honda_cup_holder_holder_v2 (Autodesk Fusion 360 design; units mm, degrees)
Autodesk Fusion 360 part; units mm, degrees
note: some values were not read from the file. Set by a fixed rule: which sketch regions a step uses.
sketch "Right Rail" plane through (0, 0, 0) normal (1, 0, 0) x (0, 0, -1)
  line L0 (7.5, 117.1) -> (11, 117.1)
  line L1 (11, 127.5) -> (16, 124.55)
  line L2 (16, 120.05) -> (11, 117.1)
  line L3 (16, 124.55) -> (16, 120.05)
  line L4 (11, 127.5) -> (7.5, 127.5)
  line L5 (7.5, 127.5) -> (7.5, 117.1)
  dimension "d1" = 5
  dimension "d2" = 4.5
  dimension "d5" = 8.5
  dimension "d16" = 10.4
  dimension "d17" = 7.5
  dimension "d18" = 127.5
  constraint equal L1 L2
  constraint perpendicular L0 L5
  constraint vertical L3
  constraint equal L0 L4
  measures "d1" distance of L1.start L3
  measures "d2" distance of L1.end L2.start
  measures "d5" distance of L3 L5
  measures "d16" distance of L0 L4
  measures "d17" horizontal distance of origin L4.end
  measures "d18" distance of origin L4
sketch "Phone Holder" plane through (0, 0, 0) normal (0, 1, 0) x (1, 0, 0)
  line L0 (0, 7.5) -> (0, -122.5)
  line L1 (0, -122.5) -> (21.5, -122.5)
  line L2 (21.5, -122.5) -> (21.5, 7.5)
  line L3 (21.5, 7.5) -> (0, 7.5)
  line L4 (2, -10) -> (19.5, -10)
  line L5 (19.5, -10) -> (19.5, -105)
  line L6 (19.5, -105) -> (2, -105)
  line L7 (2, -105) -> (2, -10)
  line L8 (2, -105) -> (2, -122.5) construction
  line L9 (2, -10) -> (2, 7.5) construction
  dimension "d6" = 2
  dimension "d7" = 2
  dimension "d8" = 17.5
  dimension "d9" = 95
  dimension "d10" = 7.5
  dimension "d11" = 130
  constraint vertical L0
  constraint perpendicular L0 L1
  constraint perpendicular L1 L2
  constraint perpendicular L2 L3
  constraint horizontal L4
  constraint vertical L5
  constraint horizontal L6
  constraint vertical L7
  constraint coincident origin L0
  constraint coincident L1 L8.end
  constraint perpendicular L1 L8
  constraint coincident L3 L9.end
  constraint perpendicular L3 L9
  constraint equal L8 L9
  measures "d6" distance of L2 L5
  measures "d7" distance of L0 L7
  measures "d8" distance of L4.start L4.end
  measures "d9" distance of L4 L6
  measures "d10" distance of L3 origin
  measures "d11" distance of L1 L3
extrude "Extrude2" add sketch "Phone Holder" along normal blind 3 contours L4 L5 L6 L7 makes body 1
extrude "Extrude1" add sketch "Phone Holder" along normal blind 130 separate body makes body 2
extrude "Extrude3" add sketch "Right Rail" along normal blind 21.5 bodies 2
sketch "Spring Rail Hole" plane through (0, 0, 122.5) normal (0, 0, 1) x (1, 0, 0)
  line L0 (0, 0) -> (21.5, 0)
  line L1 (21.5, 0) -> (21.5, 130)
  line L2 (21.5, 130) -> (0, 130)
  line L3 (0, 130) -> (0, 0)
  line L4 (2.5, 127.5) -> (2.5, 116.9)
  line L5 (19, 116.9) -> (19, 127.5)
  line L6 (19, 127.5) -> (2.5, 127.5)
  line L7 (2.5, 116.9) -> (9.375, 116.9)
  line L8 (9.375, 116.9) -> (9.375, 113.9)
  line L9 (9.375, 113.9) -> (12.125, 113.9)
  line L10 (12.125, 113.9) -> (12.125, 116.9)
  line L11 (12.125, 116.9) -> (19, 116.9)
  dimension "d21" = 2.5
  dimension "d23" = 2.5
  dimension "d24" = 2.5
  dimension "d27" = 2.75
  dimension "d29" = 3
  dimension "d30" = 10.6
  constraint parallel L3 L4
  constraint horizontal L6
  constraint perpendicular L4 L7
  constraint perpendicular L7 L8
  constraint perpendicular L4 L9
  constraint perpendicular L9 L10
  constraint equal L7 L11
  constraint coincident L5.start L11.end
  constraint perpendicular L5 L11
  constraint collinear L7 L11
  measures "d21" distance of L2 L6
  measures "d23" distance of L1 L5
  measures "d24" distance of L3 L4
  measures "d27" distance of L8.end L9.end
  measures "d29" distance of L9.end L10.end
  measures "d30" distance of L5.start L5.end
extrude "Extrude4" cut sketch "Spring Rail Hole" against normal blind 15 contours L4 L5 L6 L7 L8 L9 L10 L11 bodies 2
sketch "Spting Cross" plane through (0, 0, 107.5) normal (0, 0, 1) x (1, 0, 0)
  line L0 (12.125, 116.9) -> (19, 116.9)
  line L1 (19, 116.9) -> (19, 127.5)
  line L2 (19, 127.5) -> (2.5, 127.5)
  line L3 (2.5, 127.5) -> (2.5, 116.9)
  line L4 (2.5, 116.9) -> (9.375, 116.9)
  line L5 (9.375, 116.9) -> (9.375, 113.9)
  line L6 (9.375, 113.9) -> (12.125, 113.9)
  line L7 (12.125, 113.9) -> (12.125, 116.9)
  line L8 (10.25, 124.7) -> (10.25, 122.7)
  line L9 (10.25, 122.7) -> (8.25, 122.7)
  line L10 (8.25, 122.7) -> (8.25, 121.7)
  line L11 (8.25, 121.7) -> (10.25, 121.7)
  line L12 (10.25, 121.7) -> (10.25, 119.7)
  line L13 (10.25, 119.7) -> (11.25, 119.7)
  line L14 (11.25, 119.7) -> (11.25, 121.7)
  line L15 (11.25, 121.7) -> (13.25, 121.7)
  line L16 (13.25, 121.7) -> (13.25, 122.7)
  line L17 (13.25, 122.7) -> (11.25, 122.7)
  line L18 (10.25, 124.7) -> (11.25, 124.7)
  line L19 (11.25, 124.7) -> (11.25, 122.7)
  line L20 (8.25, 122.2) -> (13.25, 122.2) construction
  line L21 (2.5, 122.2) -> (19, 122.2) construction
  dimension "d31" = 1
  dimension "d32" = 5
  constraint perpendicular L2 L8
  constraint perpendicular L8 L9
  constraint perpendicular L9 L10
  constraint perpendicular L10 L11
  constraint perpendicular L11 L12
  constraint perpendicular L12 L13
  constraint perpendicular L13 L14
  constraint perpendicular L14 L15
  constraint perpendicular L15 L16
  constraint perpendicular L16 L17
  constraint perpendicular L8 L18
  constraint perpendicular L17 L19
  constraint equal L8 L19
  constraint equal L9 L17
  constraint equal L8 L12
  constraint equal L11 L15
  constraint equal L8 L9
  constraint equal L14 L15
  constraint equal L13 L18
  constraint equal L16 L18
  constraint midpoint L10 L20.start
  constraint midpoint L16 L20.end
  constraint midpoint L3 L21.start
  constraint midpoint L1 L21.end
  constraint midpoint L20 L21
  measures "d31" distance of L8.start L18.end
  measures "d32" distance of L10 L16
extrude "Extrude5" add sketch "Spting Cross" along normal blind 7.5 contours L8 L9 L10 L11 L12 L13 L14 L15 L16 L17 L18 L19 bodies 2
sketch "Phone Holder Hole" plane through (21.5, 0, 0) normal (1, 0, 0) x (0, 0, -1)
  line L0 (-122.5, 0) -> (7.5, 0)
  line L1 (7.5, 0) -> (7.5, 117.1)
  line L2 (7.5, 117.1) -> (11, 117.1)
  line L3 (11, 117.1) -> (16, 120.05)
  line L4 (16, 120.05) -> (16, 124.55)
  line L5 (16, 124.55) -> (11, 127.5)
  line L6 (11, 127.5) -> (7.5, 127.5)
  line L7 (7.5, 127.5) -> (7.5, 130)
  line L8 (7.5, 130) -> (-122.5, 130)
  line L9 (-122.5, 130) -> (-122.5, 0)
  line L10 (-72.5, 130) -> (-72.5, 70)
  arc A0 (-72.5, 70) -> (-42.5, 70) centre (-57.5, 70) ccw
  line L11 (-42.5, 70) -> (-42.5, 130)
  line L12 (-122.5, 130) -> (-72.5, 130) construction
  line L13 (-42.5, 130) -> (7.5, 130) construction
  circle A1 centre (-97.5, 25) radius 12.5
  circle A2 centre (-17.5, 25) radius 12.5
  circle A3 centre (-57.5, 25) radius 12.5
  line L14 (-122.5, 25) -> (7.5, 25) construction
  line L15 (-122.5, 0) -> (7.5, 0) construction
  line L16 (-57.5, 70) -> (-57.5, 25) construction
  line L17 (-97.5, 25) -> (-97.5, 70) construction
  line L18 (-17.5, 25) -> (-17.5, 70) construction
  line L19 (-17.5, 70) -> (-97.5, 70) construction
  circle A4 centre (-97.5, 70) radius 53.4439 construction
  circle A5 centre (-97.5, 70) radius 12.5
  circle A6 centre (-17.5, 70) radius 12.5
  line L20 (-97.5, 70) -> (-97.5, 102.4132) construction
  line L21 (-17.5, 101.7961) -> (-97.5, 102.4132) construction
  line L22 (-17.5, 101.7961) -> (-17.5, 70) construction
  circle A7 centre (-97.5, 102.4132) radius 13.0731 construction
  circle A8 centre (-17.5, 101.7961) radius 13.7934 construction
  dimension "d35" = 30
  dimension "d36" = 60
  dimension "d47" = 40
  dimension "d48" = 40
  dimension "d49" = 25
  dimension "d50" = 25
  dimension "d51" = 25
  dimension "d52" = 25
  dimension "d53" = 25
  dimension "d54" = 25
  dimension "d55" = 45
  constraint coincident L8 L10.start
  constraint perpendicular L8 L10
  constraint tangent L10 A0
  constraint coincident L8 L11.end
  constraint tangent A0 L11
  constraint perpendicular L8 L11
  constraint coincident L8.end L9.start
  constraint coincident L7.end L8.start
  constraint equal L12 L13
  constraint coincident L9 L14.start
  constraint coincident L1 L14.end
  constraint perpendicular L1 L14
  constraint coincident A1.centre L14
  constraint coincident A3.centre L14
  constraint coincident A2.centre L14
  constraint coincident A0.centre L16.start
  constraint midpoint L14 A3.centre
  constraint coincident A3.centre L16.end
  constraint coincident A1.centre L17.start
  constraint perpendicular L14 L17
  constraint coincident A2.centre L18.start
  constraint perpendicular L14 L18
  constraint perpendicular L17 L19
  constraint coincident L17.end L19.end
  constraint coincident L18.end L19.start
  constraint perpendicular L19 L20
  constraint perpendicular L19 L22
  constraint coincident L20.end L21.end
  constraint coincident L21.start L22.start
  measures "d35" distance of L10 L11
  measures "d36" vertical distance of A0.centre L11.end
  measures "d47" distance of A1.centre A3.centre
  measures "d48" distance of A2.centre A3.centre
  measures "d49" diameter of A1
  measures "d50" diameter of A3
  measures "d51" diameter of A2
  measures "d52" distance of L14.start L15
  measures "d53" diameter of A5
  measures "d54" diameter of A6
  measures "d55" distance of L14 L19
extrude "Extrude6" cut sketch "Phone Holder Hole" against normal blind 21.5 contours L8 L10 A0 L11 | A1 | A2 | A3 | A5 | A6 bodies 2
sketch "Sketch6" plane through (2.5, 0, 0) normal (1, 0, 0) x (0, 0, -1)
  line L0 (-122.5, 127.5) -> (-122.5, 116.9)
  line L1 (-122.5, 116.9) -> (-107.5, 116.9)
  line L2 (-107.5, 116.9) -> (-107.5, 127.5)
  line L3 (-107.5, 127.5) -> (-122.5, 127.5)
  line L4 (-119.5, 127.5) -> (-119.5, 116.9)
  line L5 (-107.5, 127.5) -> (-119.5, 127.5)
  line L6 (-107.5, 116.9) -> (-119.5, 116.9)
  dimension "d41" = 3
  constraint coincident L3 L4.start
  constraint coincident L1 L4.end
  constraint perpendicular L1 L4
  constraint coincident L1 L2.start
  constraint coincident L3 L2.end
  constraint coincident L2.end L3.start
  constraint coincident L1.end L2.start
  measures "d41" distance of L0 L4
extrude "Extrude7" cut sketch "Sketch6" against normal blind 1.5 contours L1 L2 L3 L4 L5 L6 bodies 2
sketch "Sketch7" plane through (19, 0, 0) normal (-1, 0, 0) x (0, 0, 1)
  line L0 (122.5, 116.9) -> (122.5, 127.5)
  line L1 (122.5, 127.5) -> (107.5, 127.5)
  line L2 (107.5, 127.5) -> (107.5, 116.9)
  line L3 (107.5, 116.9) -> (122.5, 116.9)
  line L4 (119.5, 116.9) -> (119.5, 127.5)
  line L5 (119.5, 127.5) -> (107.5, 127.5)
  line L6 (119.5, 116.9) -> (107.5, 116.9)
  dimension "d44" = 3
  constraint coincident L3 L4.start
  constraint coincident L1 L4.end
  constraint perpendicular L1 L4
  constraint coincident L1 L2.start
  constraint coincident L3 L2.end
  constraint coincident L1.end L2.start
  constraint coincident L2.end L3.start
  measures "d44" distance of L0.end L4.end
extrude "Extrude8" cut sketch "Sketch7" against normal blind 1.5 contours L1 L2 L3 L4 L5 L6 bodies 2
equation "d10 = 16 mm - 8.5 mm"
equation "d17 = 16 mm - 8.5 mm"
equation "d18 = 130 mm - 2.5 mm"
